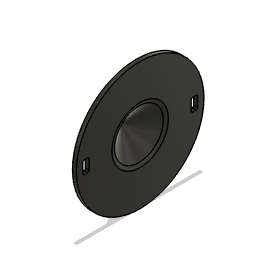
mirror_attachement (Autodesk Fusion 360 design; units mm, degrees)
Autodesk Fusion 360 part; units mm, degrees
sketch "Sketch1" plane through (0, 0, 0) normal (0, 1, 0) x (1, 0, 0)
  line L0 (0, 0) -> (0, 23.75)
  line L1 (0, 0) -> (0, 50)
  line L2 (0, 50) -> (3, 50)
  line L3 (3, 50) -> (3, 0)
  line L4 (0, 0) -> (-16.0313, 0)
  line L5 (0, 23.75) -> (-16.0313, 0)
  line L6 (3, 0) -> (0, 0)
  dimension "d1" = 23.75
  dimension "d2" = 3
  dimension "d3" = 16.0313
  constraint coincident L0.start L1.start
  constraint vertical L0
  constraint parallel L0 L1
  constraint perpendicular L0 L2
  constraint perpendicular L2 L3
  constraint perpendicular L1 L4
  constraint perpendicular L0 L6
  measures "d1" distance of L0.start L0.end
  measures "d2" distance of L1.end L2.end
  measures "d3" distance of L0.start L4.end
revolve "Revolve1" add sketch "Sketch1" angle 360 about axis through (0, 0, 0) along (-1, 0, 0) contours L0 L1 L4 L5
revolve "Revolve2" add sketch "Sketch1" angle 360 about axis through (3, 0, 0) along (-1, 0, 0) contours L0 L1 L2 L3 L6
sketch "Sketch2" plane through (0, 0, 0) normal (0, 1, 0) x (1, 0, 0)
  line L0 (0, 0) -> (3, 0)
  line L1 (3, 0) -> (-12, 0)
  line L2 (3, 0) -> (3, 20.5)
  line L3 (3, 20.5) -> (-12, 0)
  line L4 (3, 20.5) -> (3, 0)
  dimension "d6" = 3
  dimension "d7" = 15
  dimension "d8" = 20.5
  constraint coincident L0.start origin
  constraint horizontal L0
  constraint parallel L0 L1
  constraint perpendicular L1 L2
  measures "d6" distance of L0.start L0.end
  measures "d7" distance of L0.end L1.end
  measures "d8" distance of L0.end L2.end
revolve "Revolve3" cut sketch "Sketch2" angle 360 about axis through (1.75, 0, 0) along (1, 0, 0)
sketch "Sketch3" plane through (3, 0, 0) normal (1, 0, 0) x (0, 0, -1)
  circle A0 centre (0, 0) radius 50
  line L0 (0, 0) -> (0, 5)
  line L1 (0, 5) -> (0, -5)
  line L2 (0, 5) -> (-45, 5)
  line L3 (0, -5) -> (-45, -5)
  line L4 (-45, 5) -> (-45, -5)
  line L5 (-45, 5) -> (-40, 5)
  line L6 (-40, 5) -> (-40, -5)
  line L7 (-40, -5) -> (-45, -5)
  line L8 (-45, -5) -> (-45, 5)
  line L9 (40, 5) -> (40, -5)
  line L10 (0, 5) -> (45, 5)
  line L11 (45, -5) -> (45, 5)
  line L12 (40, -5) -> (45, -5)
  line L13 (0, -5) -> (45, -5)
  circle A1 centre (0, 0) radius 20.5
  dimension "d16" = 5
  dimension "d17" = 10
  dimension "d18" = 45
  dimension "d19" = 5
  constraint coincident A0.centre L0.start
  constraint vertical L0
  constraint parallel L0 L1
  constraint perpendicular L0 L2
  constraint perpendicular L1 L3
  constraint horizontal L5
  constraint vertical L6
  constraint horizontal L7
  constraint vertical L8
  constraint symmetric L0.end L1 L2.start
  constraint symmetric L3.start L1 L13.start
  constraint symmetric L1 L2.end L10.end
  constraint symmetric L1 L3.end L11.start
  constraint symmetric L1 L5.end L9.start
  constraint symmetric L1 L6.end L9.end
  measures "d16" distance of A0.centre L0.end
  measures "d17" distance of L0.end L1.end
  measures "d18" distance of L1.end L3.end
  measures "d19" distance of L2.end L5.end
extrude "Extrude2" cut sketch "Sketch3" against normal blind 3 contours L2 L3 L4 L5 L6 L7 L8 | L9 L10 L11 L12 L13
fillet "Fillet2" radius 1 8 edges at (1.5, 5, 45) (1.5, 5, 40) (1.5, -5, 40) (1.5, -5, 45) (1.5, 5, -45) (1.5, 5, -40) (1.5, -5, -40) (1.5, -5, -45)
fillet "Fillet3" radius 5 1 edges at (3, 7.4131, 19.1127)
equation "d1 = ( 47.5 / 2 ) * 1 mm"
equation "d3 = ( 1.60313 * 10 ) * 1 mm"
equation "d7 = 18.000 mm - 3 mm"
equation "d8 = 23.5 mm - 3 mm"
